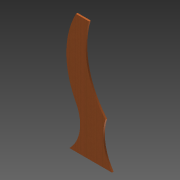
# Autodesk Inventor part: side
Saved by Autodesk Inventor 2013 (Build 170138000, 138)
## iProperties
Created: 2013-05-02
Part Number: side
Material: Wood (Cherry)
Document SubType Name: Modeling
Designer: Chris
Density: 1 g/cm^3
Author: Chris
Autodesk Inventor part; units mm, degrees
ref_plane "YZ Plane" through (0, 0, 0) normal (1, 0, 0) x (0, 1, 0)
ref_plane "XZ Plane" through (0, 0, 0) normal (0, 1, 0) x (-1, 0, 0)
ref_plane "XY Plane" through (0, 0, 0) normal (0, 0, 1) x (1, 0, 0)
sketch "Sketch1" plane through (0, 0, 0) normal (0, 0, 1) x (1, 0, 0)
  line L0 (0, 0) -> (457.2, 0)
  line L1 (0, 1192.4482) -> (0, 0)
  arc A0 (0, 1192.4482) -> (0, 0) centre (1121.346, 596.2241) ccw
  arc A1 (203.2, 1192.4482) -> (457.2, 0) centre (1419.8846, 828.3347) ccw
  line L2 (0, 0) -> (508.1314, 0)
  line L3 (0, 0) -> (-101.6, -660.4)
  line L4 (-101.6, -660.4) -> (558.8, -660.4)
  line L5 (558.8, -660.4) -> (457.2, 0)
  arc A2 (-101.6, -660.4) -> (0, 0) centre (-493.0572, -262.1604) ccw
  arc A3 (457.2, 0) -> (558.8, -660.4) centre (1184.8949, -226.0623) ccw
  line L6 (203.2, 1192.4482) -> (457.2, 0)
  line L7 (203.2, 1192.4482) -> (0, 1192.4482)
  dimension "d0" = 457.2
  dimension "d1" = 1219.2
  dimension "d2" = 1270
  dimension "d5" = 660.4
  dimension "d6" = 660.4
  dimension "d7" = 762
  dimension "d10" = 203.2
  constraints: 16 end point, 8 point on circle, 4 centre point, 3 horizontal, 1 equal length, 1 equal radius, 1 parallel, 1 tangent, 1 vertical
  measures "d0" distance of L0.start L0.end
  measures "d1" distance of L0.end L6.start
  measures "d2" radius of A0
  measures "d5" distance of L3.end L4.end
  measures "d6" distance between parallel lines of L0 L4
  measures "d7" radius of A3
  measures "d10" distance of L6.start L1.start
extrude "Extrusion1" add sketch "Sketch1" along normal blind 25.4 contours L1 L7 A1 L0 | A0 L1 | L0 A3 L4 A2
body "Solid1"
